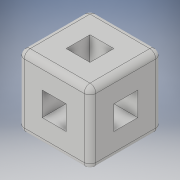
# Autodesk Inventor part: cube practice
Saved by Autodesk Inventor 2017 (Build 210142000, 142)
## iProperties
Created: 2018-09-24
Part Number: cube practice
Material: Generic
Document SubType Name: Modeling
Designer: qthuynh
Density: 1 g/cm^3
Appearance: Default
Author: qthuynh
Autodesk Inventor part; units mm, degrees
ref_plane "YZ Plane" through (0, 0, 0) normal (1, 0, 0) x (0, 1, 0)
ref_plane "XZ Plane" through (0, 0, 0) normal (0, 1, 0) x (-1, 0, 0)
ref_plane "XY Plane" through (0, 0, 0) normal (0, 0, 1) x (1, 0, 0)
sketch "Sketch1" plane through (0, 0, 0) normal (0, 0, 1) x (1, 0, 0)
  line L0 (0, 0) -> (152.4, 0)
  line L1 (152.4, 0) -> (152.4, 152.4)
  line L2 (152.4, 152.4) -> (0, 152.4)
  line L3 (0, 152.4) -> (0, 0)
  dimension "d0" = 152.4
  dimension "d1" = 152.4
  constraints: 8 end point, 2 parallel, 1 horizontal, 1 perpendicular
  measures "d0" distance of L2.end L1.end
  measures "d1" distance of L1.end L0.end
extrude "Extrusion1" add sketch "Sketch1" along normal blind 152.4
sketch "Sketch2" plane through (0, 0, 152.4) normal (0, 0, 1) x (1, 0, 0)
  line L0 (50.8, 50.8) -> (101.6, 50.8)
  line L1 (101.6, 50.8) -> (101.6, 101.6)
  line L2 (101.6, 101.6) -> (50.8, 101.6)
  line L3 (50.8, 101.6) -> (50.8, 50.8)
  line L4 (152.4, 152.4) -> (0, 152.4) projected
  line L5 (152.4, 0) -> (152.4, 152.4) projected
  point P0 (0, 0)
  dimension "d4" = 50.8
  dimension "d5" = 50.8
  dimension "d6" = 50.8
  dimension "d7" = 50.8
  constraints: 8 end point, 2 parallel, 1 horizontal, 1 perpendicular
  measures "d4" distance of L2.end L1.end
  measures "d5" distance of L1.end L0.end
  measures "d6" distance from line of L4 L2.end
  measures "d7" distance from line of L5 L1.end
extrude "Extrusion2" cut sketch "Sketch2" against normal blind 182.5625
sketch "Sketch3" plane through (152.4, 0, 0) normal (1, 0, 0) x (0, 0, -1)
  line L0 (-101.6, 50.8) -> (-50.8, 50.8)
  line L1 (-50.8, 50.8) -> (-50.8, 101.6)
  line L2 (-50.8, 101.6) -> (-101.6, 101.6)
  line L3 (-101.6, 101.6) -> (-101.6, 50.8)
  line L4 (0, 152.4) -> (-152.4, 152.4) projected
  line L5 (-152.4, 0) -> (-152.4, 152.4) projected
  point P0 (0, 0)
  dimension "d10" = 50.8
  dimension "d11" = 50.8
  dimension "d12" = 50.8
  dimension "d13" = 50.8
  constraints: 8 end point, 2 parallel, 1 horizontal, 1 perpendicular
  measures "d10" distance of L2.end L1.end
  measures "d11" distance of L1.end L0.end
  measures "d12" distance from line of L4 L1.end
  measures "d13" distance from line of L5 L2.end
extrude "Extrusion3" cut sketch "Sketch3" against normal blind 182.5625
sketch "Sketch4" plane through (0, 152.4, 0) normal (0, 1, 0) x (1, 0, 0)
  line L0 (101.6, -101.6) -> (50.8, -101.6)
  line L1 (50.8, -101.6) -> (50.8, -50.8)
  line L2 (50.8, -50.8) -> (101.6, -50.8)
  line L3 (101.6, -50.8) -> (101.6, -101.6)
  line L4 (152.4, -152.4) -> (0, -152.4) projected
  line L5 (0, 0) -> (0, -152.4) projected
  dimension "d16" = 50.8
  dimension "d17" = 50.8
  dimension "d18" = 50.8
  dimension "d19" = 50.8
  constraints: 8 end point, 2 parallel, 1 horizontal, 1 perpendicular
  measures "d16" distance of L1.end L2.end
  measures "d17" distance of L0.end L1.end
  measures "d18" distance from line of L4 L0.end
  measures "d19" distance from line of L5 L1.end
extrude "Extrusion4" cut sketch "Sketch4" against normal blind 182.5625
fillet "Fillet1" radius 12.7 12 edges at (76.2, 152.4, 152.4) (152.4, 152.4, 76.2) (0, 76.2, 152.4) (76.2, 0, 152.4) (152.4, 0, 76.2) (152.4, 76.2, 152.4) (152.4, 76.2, 0) (0, 152.4, 76.2) (76.2, 152.4, 0) (0, 0, 76.2) (0, 76.2, 0) (76.2, 0, 0)
body "Solid1"
